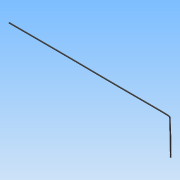
# Autodesk Inventor part: Top_Pipe Cable 2
Saved by Autodesk Inventor 2018.1 (Build 221171000, 171)
## iProperties
Created: 2019-03-23
Part Number: Top_Pipe Cable 2
Material: PVC-Piping
Document SubType Name: Modeling
Designer: James
Density: 1.4 g/cm^3
Appearance: Smooth - Black
Author: James
Autodesk Inventor part; units mm, degrees
ref_plane "YZ Plane" through (0, 0, 0) normal (1, 0, 0) x (0, 1, 0)
ref_plane "XZ Plane" through (0, 0, 0) normal (0, 1, 0) x (-1, 0, 0)
ref_plane "XY Plane" through (0, 0, 0) normal (0, 0, 1) x (1, 0, 0)
sketch "Sketch1" plane through (0, 0, 0) normal (0, 0, 1) x (1, 0, 0)
  circle A0 centre (0, 0) radius 3
  circle A1 centre (0, 0) radius 5
  dimension "d0" = 6
  dimension "d1" = 10
  constraints: 2 centre point, 2 coincident
  measures "d0" diameter of A0
  measures "d1" diameter of A1
extrude "Extrusion1" add sketch "Sketch1" against normal blind 20
sketch "Sketch4" plane through (0, 0, 0) normal (0, 0, 1) x (1, 0, 0)
  circle A0 centre (0, 0) radius 3 projected
  circle A1 centre (0, 0) radius 5 projected
sketch3d "3D Sketch1"
  spline S0 degree 4 poles (0, 0, 0) (0, 0, 172.5) (0, -5, 172.5) (0, -5, 282.5) (0, -5, 302.5) (-20, -5, 302.5) (-800.2, -5, 302.5) (-800.2, 0, 302.5) (-1450.2, 0, 302.5) knots 1 1 1 1 1 2 3 4 5 6 6 6 6 6
  dimension "d8" = 172.5
  dimension "d11" = 20
  dimension "d12" = 20
  dimension "d13" = 110
  dimension "d14" = 780.2
  dimension "d15" = 650
  dimension "d20" = 5
  dimension "d21" = 5
sweep "Sweep2" add profiles "Sketch4" path "3D Sketch1"
sketch "Sketch5" plane through (-1450.2, 0, 302.5) normal (-1, 0, 0) x (0, 0, 1)
  spline S0 degree 6 poles (3, -0.0004) (2.9993, -4.985) (-3.1644, -5.6999) (-8.2474, 0.0011) (-3.1629, 5.7008) (3.0007, 4.9842) (3, -0.0004) knots 0 0 0 0 0 0 0 1 1 1 1 1 1 1 weights 1.669078 1.03673 1.038347 0.853534 1.038347 1.03673 1.669078 projected
  circle A0 centre (0, 0) radius 5 projected
  point P0 (-302.5, 0)
  point P1 (5, -0.0004)
  constraints: 2 other
extrude "Extrusion2" add sketch "Sketch5" along normal blind 10
equation "\"d12\" = d11"
body "Solid1"
